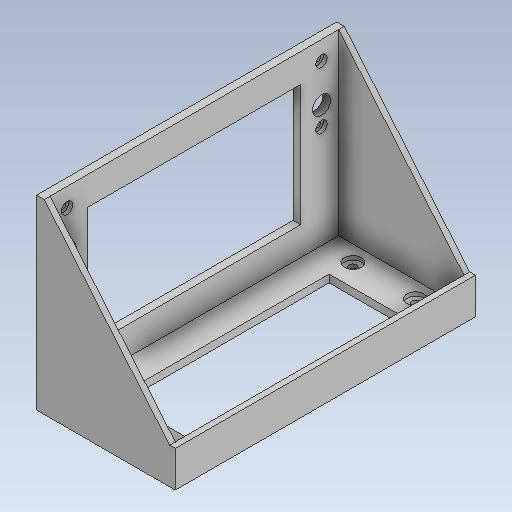
# Autodesk Inventor part: battery_box
Saved by Autodesk Inventor 2021 (Build 250183000, 183)
## iProperties
Created: 2021-03-02
Part Number: battery_box
Material: Generic
Document SubType Name: Modeling
Designer: Mateusz
Density: 1 g/cm^3
Appearance: Default
Author: Mateusz
Autodesk Inventor part; units mm, degrees
ref_plane "YZ Plane" through (0, 0, 0) normal (1, 0, 0) x (0, 1, 0)
ref_plane "XZ Plane" through (0, 0, 0) normal (0, 1, 0) x (-1, 0, 0)
ref_plane "XY Plane" through (0, 0, 0) normal (0, 0, 1) x (1, 0, 0)
sketch "Sketch1" plane through (0, 0, 0) normal (0, 1, 0) x (-1, 0, 0)
  line L0 (0, 0) -> (0, -152)
  line L1 (0, -152) -> (66, -152)
  line L2 (66, -152) -> (66, 0)
  line L3 (66, 0) -> (0, 0)
  line L4 (66, 0) -> (66, 3)
  line L5 (66, 3) -> (0, 3)
  line L6 (0, 3) -> (0, 0)
  line L7 (66, -152) -> (66, -155)
  line L8 (66, -155) -> (0, -155)
  line L9 (0, -155) -> (0, -152)
  line L10 (66, -155) -> (70, -155)
  line L11 (70, -155) -> (70, 3)
  line L12 (70, 3) -> (66, 3)
  dimension "d0" = 152
  dimension "d1" = 66
  dimension "d2" = 3
  dimension "d3" = 3
  dimension "d4" = 4
  constraints: 26 end point, 9 perpendicular, 4 point on line, 1 horizontal, 1 vertical
  measures "d0" distance of L0.start L0.end
  measures "d1" distance of L0.end L1.end
  measures "d2" distance of L2.end L4.end
  measures "d3" distance of L1.end L7.end
  measures "d4" distance of L7.end L10.end
extrude "Extrusion1" add sketch "Sketch1" against normal blind 4
extrude "Extrusion2" add sketch "Sketch1" along normal blind 94 contours L4 L12 L11 L10 L7 L2
sketch "Sketch7" plane through (0, 0, 0) normal (0, 1, 0) x (1, 0, 0)
  line L0 (0, 155) -> (0, -3) projected
  line L1 (0, -3) -> (3, -3)
  line L2 (3, -3) -> (3, 155)
  line L3 (3, 155) -> (0, 155)
  line L4 (0, 155) -> (0, -3)
  point P0 (0, 0)
  dimension "d15" = 3
  constraints: 8 end point, 2 perpendicular, 1 horizontal, 1 parallel
  measures "d15" distance of L0.end L1.end
extrude "Extrusion3" add sketch "Sketch7" against normal up to surface (4 mm away)
extrude "Extrusion4" add sketch "Sketch7" along normal blind 15
sketch "Sketch8" plane through (-66, 94, -155) normal (0, 0, -1) x (-1, 0, 0)
  line L0 (-66, -79) -> (0, 0)
  line L1 (0, -94) -> (0, 0) projected
  line L2 (0, 0) -> (0, -94)
  line L3 (-66, -94) -> (0, -94) projected
  line L4 (0, -94) -> (-66, -94)
  line L5 (-66, -94) -> (-66, -79)
  constraints: 8 end point, 2 collinear, 1 perpendicular
extrude "Extrusion5" add sketch "Sketch8" against normal blind 3
sketch "Sketch9" plane through (-70, 94, 3) normal (0, 0, 1) x (1, 0, 0)
  line L0 (0, 0) -> (4, 0) projected
  line L1 (70, -94) -> (70, -79) projected
  line L2 (4, 0) -> (70, -79)
  line L3 (70, -79) -> (70, -94)
  line L4 (4, -94) -> (70, -94) projected
  line L5 (70, -94) -> (4, -94)
  line L6 (4, -94) -> (4, 0) projected
  line L7 (4, -94) -> (4, 0)
  constraints: 8 end point, 2 collinear, 1 perpendicular
extrude "Extrusion6" add sketch "Sketch9" against normal blind 3
sketch "Sketch10" plane through (0, 0, 0) normal (0, 1, 0) x (1, 0, 0)
  line L0 (-66, 0) -> (-66, 152) projected
  line L1 (-66, 0) -> (-66, 20)
  line L2 (-66, 20) -> (-51, 20)
  line L3 (-66, 0) -> (0, 0) projected
  line L4 (0, 0) -> (0, 20)
  line L5 (0, 152) -> (0, 0) projected
  line L6 (0, 20) -> (-15, 20)
  line L7 (0, 152) -> (0, 132)
  line L8 (0, 132) -> (-15, 132)
  line L9 (0, 152) -> (-66, 152) projected
  line L10 (-66, 152) -> (-66, 132)
  line L11 (-66, 132) -> (-51, 132)
  line L12 (-51, 132) -> (-51, 20)
  line L13 (-15, 20) -> (-51, 20)
  line L14 (-15, 20) -> (-15, 132)
  line L15 (-51, 132) -> (-15, 132)
  dimension "d24" = 20
  dimension "d25" = 15
  dimension "d26" = 20
  dimension "d27" = 15
  dimension "d28" = 20
  dimension "d29" = 20
  dimension "d30" = 15
  constraints: 24 end point, 5 perpendicular, 4 point on line
  measures "d24" distance of L0.start L1.end
  measures "d25" distance of L1.end L2.end
  measures "d26" distance of L3.end L4.end
  measures "d27" distance of L4.end L6.end
  measures "d28" distance of L5.start L7.end
  measures "d29" distance of L0.end L10.end
  measures "d30" distance of L10.end L11.end
extrude "Extrusion7" cut sketch "Sketch10" against normal up to surface (4 mm away) contours L12 L15 L14 L13
sketch "Sketch11" plane through (-66, 0, -152) normal (1, 0, 0) x (0, 0, -1)
  line L0 (-152, 94) -> (0, 94) projected
  line L1 (-152, 94) -> (-132, 94)
  line L2 (-132, 94) -> (-132, 79)
  line L3 (0, 94) -> (-20, 94)
  line L4 (-20, 94) -> (-20, 79)
  line L5 (-20, 79) -> (-132, 79)
  line L6 (0, 0) -> (-152, 0) projected
  line L7 (-152, 0) -> (-132, 0)
  line L8 (-132, 0) -> (-132, 15)
  line L9 (-132, 15) -> (-132, 79)
  line L10 (0, 0) -> (-20, 0)
  line L11 (-20, 0) -> (-20, 15)
  line L12 (-20, 15) -> (-20, 79)
  line L13 (-20, 15) -> (-132, 15)
  dimension "d33" = 20
  dimension "d34" = 15
  dimension "d35" = 20
  dimension "d36" = 15
  dimension "d37" = 20
  dimension "d38" = 15
  dimension "d39" = 20
  dimension "d40" = 15
  constraints: 24 end point, 4 perpendicular, 4 point on line
  measures "d33" distance of L0.start L1.end
  measures "d34" distance of L1.end L2.end
  measures "d35" distance of L0.end L3.end
  measures "d36" distance of L3.end L4.end
  measures "d37" distance of L6.end L7.end
  measures "d38" distance of L7.end L8.end
  measures "d39" distance of L6.start L10.end
  measures "d40" distance of L10.end L11.end
extrude "Extrusion8" cut sketch "Sketch11" against normal up to surface (4 mm away) contours L5 L12 L13 L9
sketch "Sketch12" plane through (0, 0, 0) normal (0, 1, 0) x (1, 0, 0)
  line L0 (-70, -3) -> (3, -3) projected
  line L1 (3, -3) -> (3, 20)
  line L2 (3, -3) -> (3, 155) projected
  line L3 (3, -3) -> (3, 8.5)
  line L4 (3, 8.5) -> (-70, 8.5)
  line L5 (3, 8.5) -> (-17, 8.5)
  line L6 (-70, 8.5) -> (-50, 8.5)
  circle A0 centre (-17, 8.5) radius 2
  circle A1 centre (-50, 8.5) radius 2
  line L7 (-70, 155) -> (3, 155) projected
  line L8 (3, 155) -> (3, 143.5)
  line L9 (3, 143.5) -> (-70, 143.5)
  line L10 (-70, 155) -> (-70, -3) projected
  line L11 (3, 143.5) -> (-17, 143.5)
  line L12 (-70, 143.5) -> (-50, 143.5)
  circle A2 centre (-17, 143.5) radius 2
  circle A3 centre (-50, 143.5) radius 2
  dimension "d43" = 23
  dimension "d44" = 11.5
  dimension "d45" = 20
  dimension "d46" = 20
  dimension "d47" = 4
  dimension "d48" = 4
  dimension "d49" = 11.5
  dimension "d50" = 20
  dimension "d51" = 20
  dimension "d52" = 4
  dimension "d53" = 4
  constraints: 18 end point, 8 point on line, 4 centre point, 4 coincident, 2 perpendicular
  measures "d43" distance of L0.end L1.end
  measures "d44" distance of L0.end L3.end
  measures "d45" distance of L3.end L5.end
  measures "d46" distance of L4.end L6.end
  measures "d47" diameter of A0
  measures "d48" diameter of A1
  measures "d49" distance of L2.end L8.end
  measures "d50" distance of L8.end L11.end
  measures "d51" distance of L9.end L12.end
  measures "d52" diameter of A2
  measures "d53" diameter of A3
extrude "Extrusion9" cut sketch "Sketch12" against normal up to surface (4 mm away) contours A1 L4 | L4 A1 | A0 L4 | L4 A0 | A3 L9 | L9 A3 | A2 L9 | L9 A2
sketch "Sketch13" plane through (-66, 0, -152) normal (1, 0, 0) x (0, 0, -1)
  circle A0 centre (-143.0001, 84.1472) radius 1.4502 projected
  circle A1 centre (-142.9999, 54.147) radius 1.4501 projected
  circle A2 centre (-9, 84.1467) radius 1.4497 projected
  circle A3 centre (-9.0001, 54.147) radius 1.4501 projected
  point P0 (-152, 0)
extrude "Extrusion10" cut sketch "Sketch13" against normal up to surface (4 mm away)
sketch "Sketch14" plane through (-66, 0, -152) normal (1, 0, 0) x (0, 0, -1)
  circle A0 centre (-9, 84.1467) radius 1.4497 projected
  line L0 (-9, 84.1467) -> (-9, 64.0437)
  circle A1 centre (-9, 64.0437) radius 4.767
  circle A2 centre (-143.0001, 84.1472) radius 1.4502 projected
  line L1 (-143.0001, 84.1472) -> (-143.0001, 64.0437)
  circle A3 centre (-143.0001, 64.0437) radius 4.767
  point P0 (-152, 0)
  dimension "d58" = 20.103
  dimension "d59" = 9.534
  constraints: 4 end point, 2 centre point, 2 coincident, 2 vertical
  measures "d58" distance of L0.start L0.end
  measures "d59" diameter of A1
extrude "Extrusion11" cut sketch "Sketch14" against normal up to surface (4 mm away) contours A1 | A3
sketch "Sketch15" plane through (0, 0, 0) normal (0, 1, 0) x (1, 0, 0)
  circle A0 centre (-50, 8.5) radius 2 projected
  circle A1 centre (-50, 8.5) radius 4.5
  circle A2 centre (-17, 8.5) radius 2 projected
  circle A3 centre (-17, 8.5) radius 4.5
  circle A4 centre (-50, 143.5) radius 2 projected
  circle A5 centre (-50, 143.5) radius 4.5
  circle A6 centre (-17, 143.5) radius 2 projected
  circle A7 centre (-17, 143.5) radius 4.5
  point P0 (0, 0)
  dimension "d68" = 9
  dimension "d69" = 9
  dimension "d70" = 9
  dimension "d71" = 9
  constraints: 4 centre point, 4 coincident
  measures "d68" diameter of A1
  measures "d69" diameter of A3
  measures "d70" diameter of A5
  measures "d71" diameter of A7
extrude "Extrusion12" cut sketch "Sketch15" against normal blind 2
sketch "Sketch16" plane through (-66, 0, -152) normal (1, 0, 0) x (0, 0, -1)
  circle A0 centre (-143.0001, 84.1472) radius 1.4502 projected
  circle A1 centre (-143.0001, 84.1472) radius 3
  circle A2 centre (-142.9999, 54.147) radius 1.4501 projected
  circle A3 centre (-142.9999, 54.147) radius 3
  circle A4 centre (-9, 84.1467) radius 1.4497 projected
  circle A5 centre (-9, 84.1467) radius 3
  circle A6 centre (-9.0001, 54.147) radius 1.4501 projected
  circle A7 centre (-9.0001, 54.147) radius 3
  point P0 (-152, 0)
  dimension "d74" = 6
  dimension "d75" = 6
  dimension "d76" = 6
  dimension "d77" = 6
  constraints: 4 centre point, 4 coincident
  measures "d74" diameter of A1
  measures "d75" diameter of A3
  measures "d76" diameter of A5
  measures "d77" diameter of A7
extrude "Extrusion13" cut sketch "Sketch16" against normal blind 2
body "Solid1"
